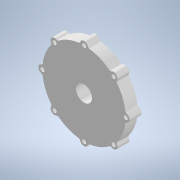
# Autodesk Inventor part: mecanum hub
Saved by Autodesk Inventor 2022 (Build 260153000, 153)
## iProperties
Created: 2022-08-08
Part Number: mecanum hub
Material: Generic
Document SubType Name: Modeling
Designer: deli
Density: 1 g/cm^3
Appearance: Default
Author: deli
Autodesk Inventor part; units mm, degrees
ref_plane "YZ Plane" through (0, 0, 0) normal (1, 0, 0) x (0, 1, 0)
ref_plane "XZ Plane" through (0, 0, 0) normal (0, 1, 0) x (-1, 0, 0)
ref_plane "XY Plane" through (0, 0, 0) normal (0, 0, 1) x (1, 0, 0)
sketch "Sketch1" plane through (0, 0, 0) normal (0, 0, 1) x (1, 0, 0)
  circle A0 centre (447.2249, 72.4085) radius 8
  circle A1 centre (447.2249, 114.2185) radius 2
  circle A2 centre (417.6608, 101.9726) radius 2
  circle A3 centre (405.4149, 72.4085) radius 2
  circle A4 centre (417.6608, 42.8443) radius 2
  circle A5 centre (447.2249, 30.5985) radius 2
  circle A6 centre (476.7891, 42.8443) radius 2
  circle A7 centre (489.0349, 72.4085) radius 2
  circle A8 centre (476.7891, 101.9726) radius 2
  circle A9 centre (447.2249, 114.2185) radius 4
  circle A10 centre (476.7891, 101.9726) radius 4
  circle A11 centre (489.0349, 72.4085) radius 4
  circle A12 centre (476.7891, 42.8443) radius 4
  circle A13 centre (447.2249, 30.5985) radius 4
  circle A14 centre (417.6608, 42.8443) radius 4
  circle A15 centre (405.4149, 72.4085) radius 4
  circle A16 centre (417.6608, 101.9726) radius 4
  circle A17 centre (447.2249, 72.4085) radius 41.81
  point P0 (0, 0)
  point P1 (443.2295, 114.0271)
  point P2 (420.6213, 104.6625)
  point P3 (414.9709, 99.0121)
  point P4 (405.6063, 76.4039)
  point P5 (405.6063, 68.413)
  point P6 (414.9709, 45.8048)
  point P7 (420.6213, 40.1544)
  point P8 (443.2295, 30.7898)
  point P9 (451.2203, 30.7898)
  point P10 (473.8286, 40.1544)
  point P11 (479.479, 45.8048)
  point P12 (488.8436, 68.413)
  point P13 (488.8436, 76.4039)
  point P14 (479.479, 99.0121)
  point P15 (473.8286, 104.6625)
  point P16 (451.2203, 114.0271)
  dimension "d0" = 16
  dimension "d1" = 4
  dimension "d4" = 360
  dimension "d6" = 32
  dimension "d7" = 8
  dimension "d8" = 8
  dimension "d9" = 8
  dimension "d10" = 8
  dimension "d11" = 8
  dimension "d12" = 8
  dimension "d13" = 8
  dimension "d14" = 8
  constraints: 17 centre point, 9 coincident, 20 other
  measures "d0" diameter of A0
  measures "d1" diameter of A1
  measures "d6" distance of A8.centre A1.centre
  measures "d7" diameter of A9
  measures "d8" diameter of A10
  measures "d9" diameter of A11
  measures "d10" diameter of A12
  measures "d11" diameter of A13
  measures "d12" diameter of A14
  measures "d13" diameter of A15
  measures "d14" diameter of A16
extrude "Extrusion1" add sketch "Sketch1" along normal blind 12 contours A1 A17 A9 | A1 A17 A9 | A9 A17 A10 A11 A12 A13 A14 A15 A16 | A17 A2 A16 | A16 A17 A2 | A17 A8 A10 | A10 A17 A8 | A17 A3 A15 | A15 A17 A3 | A17 A7 A11 | A11 A17 A7 | A17 A4 A14 | A14 A17 A4 | A17 A6 A12 | A12 A17 A6 | A17 A5 A13 | A13 A17 A5
fillet "Fillet1" radius 2 16 edges at (451.2203, 114.0271, 6) (479.479, 99.0121, 6) (473.8286, 104.6625, 6) (488.8436, 76.4039, 6) (488.8436, 68.413, 6) (479.479, 45.8048, 6) (420.6213, 104.6625, 6) (443.2295, 114.0271, 6) (414.9709, 99.0121, 6) (405.6063, 76.4039, 6) (414.9709, 45.8048, 6) (405.6063, 68.413, 6) (420.6213, 40.1544, 6) (443.2295, 30.7898, 6) (473.8286, 40.1544, 6) (451.2203, 30.7898, 6)
equation "\"d8\" = d7"
equation "\"d9\" = d7"
equation "\"d10\" = d7"
equation "\"d11\" = d7"
equation "\"d12\" = d7"
equation "\"d13\" = d7"
equation "\"d14\" = d7"
body "Solid1"
